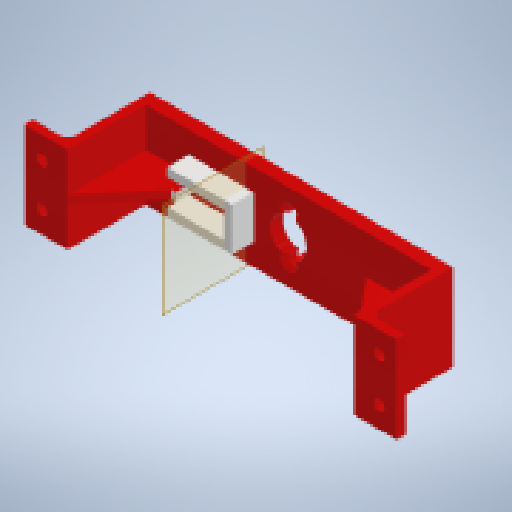
# Autodesk Inventor part: Soporte motor
Saved by Autodesk Inventor 2023 (Build 270158000, 158)
## iProperties
Created: 2022-12-05
Part Number: Soporte motor
Material: Genérico
Document SubType Name: Modeling
Designer: sergi
Density: 1 g/cm^3
Appearance: Valor por defecto
Author: sergi
Autodesk Inventor part; units mm, degrees
ref_plane "XZ Plane" through (0, 0, 0) normal (0, 1, 0) x (-1, 0, 0)
ref_plane "XY Plane" through (0, 0, 0) normal (0, 0, 1) x (1, 0, 0)
sketch "Boceto1" plane through (0, 0, 0) normal (0, 0, 1) x (1, 0, 0)
  circle A0 centre (0, 0) radius 4.25
  line L0 (-35, -10) -> (35, -10)
  line L1 (35, -10) -> (35, 10)
  line L2 (35, 10) -> (-35, 10)
  line L3 (-35, 10) -> (-35, -10)
  line L4 (-35, -10) -> (35, 10) construction
  line L5 (35, -10) -> (-35, 10) construction
  circle A1 centre (0, 0) radius 8
  dimension "d0" = 8.5
  dimension "d1" = 70
  dimension "d2" = 20
  dimension "d3" = 16
  constraints: 12 end point, 2 centre point, 2 coincident, 2 midpoint, 2 parallel, 1 horizontal, 1 perpendicular
  measures "d0" diameter of A0
  measures "d1" distance of L2.end L1.end
  measures "d2" distance of L1.end L0.end
  measures "d3" diameter of A1
extrude "Extrusión1" add sketch "Boceto1" along normal blind 3 contours L3 L2 L1 L0 | A1
sketch "Boceto3" plane through (0, 0, 3) normal (0, 0, 1) x (1, 0, 0)
  line L0 (-35, 10) -> (-35, -10) projected
  line L1 (-35, -10) -> (-33, -10)
  line L2 (-33, -10) -> (-33, 10)
  line L3 (-33, 10) -> (-35, 10)
  line L4 (-35, 10) -> (-35, -10)
  line L5 (35, -10) -> (33, -10)
  line L6 (33, -10) -> (33, 10)
  line L7 (33, 10) -> (35, 10)
  line L8 (35, 10) -> (35, -10)
  point P0 (0, 0)
  dimension "d10" = 2
  dimension "d11" = 20
  dimension "d12" = 2
  dimension "d13" = 20
  constraints: 16 end point, 4 parallel, 2 horizontal, 2 perpendicular, 1 point on line
  measures "d10" distance of L3.end L2.end
  measures "d11" distance of L2.end L1.end
  measures "d12" distance of L6.end L7.end
  measures "d13" distance of L5.end L6.end
ref_plane "Plano de trabajo1" through (-48.5042, -32, 20) normal (0, 0, -1) x (0, 1, 0)
extrude "Extrusión3" add sketch "Boceto3" along normal blind 18
sketch "Boceto4" plane through (0, 0, 3) normal (0, 0, 1) x (1, 0, 0)
  circle A0 centre (0, 0) radius 4.25 projected
  circle A1 centre (0, -5) radius 1 projected
  circle A2 centre (0, 5) radius 1 projected
hole "Agujero1" at (0, -5, 3) at (0, 5, 3) direction (0, 0, -1) diameter 2 depth 3
chamfer "Chaflán1" distance 1 angle 45 2 edges at (0, 6, 3) (0, -6, 3)
sketch "Boceto5" plane through (-35, -10, 0) normal (-1, 0, 0) x (0, 0, 1)
  line L0 (0, 0) -> (21, 0) projected
  line L1 (21, 0) -> (19, 0)
  line L2 (19, 0) -> (19, 20)
  line L3 (19, 20) -> (21, 20)
  line L4 (21, 20) -> (21, 0)
  point P0 (0, 10)
  dimension "d49" = 2
  dimension "d50" = 20
  constraints: 8 end point, 2 parallel, 1 horizontal, 1 perpendicular
  measures "d49" distance of L2.end L3.end
  measures "d50" distance of L1.end L2.end
extrude "Extrusión4" add sketch "Boceto5" along normal blind 8
sketch "Boceto6" plane through (35, -10, 0) normal (1, 0, 0) x (0, 0, -1)
  line L0 (0, 20) -> (-21, 20) projected
  line L1 (-21, 20) -> (-19, 20)
  line L2 (-19, 20) -> (-19, 0)
  line L3 (-19, 0) -> (-21, 0)
  line L4 (-21, 0) -> (-21, 20)
  point P0 (0, 10)
  dimension "d51" = 2
  dimension "d52" = 20
  constraints: 8 end point, 2 parallel, 1 horizontal, 1 perpendicular
  measures "d51" distance of L2.end L3.end
  measures "d52" distance of L1.end L2.end
extrude "Extrusión5" add sketch "Boceto6" along normal blind 8
sketch "Boceto8" plane through (0, 0, 21) normal (0, 0, 1) x (1, 0, 0)
  line L0 (43, 10) -> (43, -10) projected
  line L1 (33, 10) -> (43, 10) projected
  line L2 (33, -10) -> (43, -10) projected
  point P0 (0, 0)
  point P1 (39, -5)
  point P2 (39, 5)
  dimension "d53" = 4
  dimension "d54" = 4
  dimension "d55" = 5
  dimension "d56" = 5
  measures "d53" distance from line of L0 point (39, -5)
  measures "d54" distance from line of L0 point (39, 5)
  measures "d55" distance from line of L1 point (39, 5)
  measures "d56" distance from line of L2 point (39, -5)
hole "Agujero3" at (39, 5, 21) at (39, -5, 21) direction (0, 0, -1) diameter 2.5 end through all
sketch "Boceto9" plane through (0, 0, 21) normal (0, 0, 1) x (1, 0, 0)
  line L0 (-33, 10) -> (-43, 10) projected
  line L1 (-43, -10) -> (-43, 10) projected
  line L2 (-33, -10) -> (-43, -10) projected
  point P0 (0, 0)
  point P1 (-39, 5)
  point P2 (-39, -5)
  dimension "d64" = 5
  dimension "d65" = 4
  dimension "d73" = 5
  dimension "d74" = 4
  measures "d64" distance from line of L0 point (-39, 5)
  measures "d65" distance from line of L1 point (-39, 5)
  measures "d73" distance from line of L2 point (-39, -5)
  measures "d74" distance from line of L1 point (-39, -5)
hole "Agujero4" at (-39, 5, 21) at (-39, -5, 21) direction (0, 0, -1) diameter 2.5 end through all
sketch "Boceto10" plane through (0, 0, 3) normal (0, 0, 1) x (1, 0, 0)
  line L0 (33, -10) -> (33, 10) projected
  line L1 (33, 0) -> (33, 1)
  line L2 (33, 0) -> (34, 0) construction
  line L3 (33, 1) -> (18, 1)
  line L4 (18, 1) -> (18, -1)
  line L5 (18, -1) -> (33, -1)
  line L6 (33, -1) -> (33, 1)
  point P0 (0, 0)
  dimension "d75" = 1
  dimension "d76" = 90
  dimension "d77" = 15
  dimension "d78" = 2
  constraints: 12 end point, 2 horizontal, 2 parallel, 2 perpendicular, 1 collinear, 1 midpoint
  measures "d75" distance of L1.start L1.end
  measures "d76" angle of L2 L1
  measures "d77" distance of L5.end L4.end
  measures "d78" distance of L4.end L3.end
extrude "Extrusión6" add sketch "Boceto10" along normal blind 18
chamfer "Chaflán2" distance 15 distance2 18 1 edges at (18, 0, 21) measured on face at (18.5, 0, 21)
fillet "Empalme2" radius 2 2 edges at (35, 0, 19) (-35, 0, 19)
mirror "Simetría1" about plane through (0, 0, 0) normal (1, 0, 0) of "Extrusión6", "Chaflán2"
ref_plane "Plano de trabajo2" through (-10, 0, 0) normal (1, 0, 0) x (0, 1, 0)
sketch "Boceto12" plane through (0, 0, 3) normal (0, 0, 1) x (1, 0, 0)
  line L0 (-10, -3) -> (-21, -3) projected
  line L1 (-21, -3) -> (-21, 3) projected
  line L2 (-10, 3) -> (-21, 3) projected
  line L3 (-10, -3) -> (-10, 3) projected
  point P0 (0, 0)
extrude "Extrusión7" cut sketch "Boceto12" along normal blind 10
sketch "Boceto13" plane through (0, 0, 3) normal (0, 0, 1) x (1, 0, 0)
  line L0 (-10, -3) -> (-21, -3) projected
  line L1 (-21, -3) -> (-21, 3) projected
  line L2 (-10, 3) -> (-21, 3) projected
  line L3 (-10, -3) -> (-10, 3) projected
  line L4 (-23, -5) -> (-8, -5)
  line L5 (-8, -5) -> (-8, 5)
  line L6 (-8, 5) -> (-23, 5)
  line L7 (-23, 5) -> (-23, -5)
  line L8 (-10, -3) -> (-8, -3)
  line L9 (-10, 3) -> (-8, 3)
  line L10 (-33, -1) -> (-21, -1) projected
  line L11 (-21, 1) -> (-33, 1) projected
  line L12 (-21, -3) -> (-23, -3)
  line L13 (-21, 3) -> (-23, 3)
  point P0 (0, 0)
  point P1 (-23, 1)
  point P2 (-23, -1)
  dimension "d88" = 2
  constraints: 16 end point, 4 point on line, 3 perpendicular, 1 parallel, 3 other
  measures "d88" distance between parallel lines of L0 L4
extrude "Extrusión8" add sketch "Boceto13" along normal blind 5 contours L8 L5 L4 L7 L12 L0 | L3 L9 L5 L8 | L2 L13 L7 L6 L5 L9
sketch "Boceto14" plane through (0, 0, 8) normal (0, 0, 1) x (1, 0, 0)
  line L0 (-10, 3) -> (-10, -3) projected
  line L1 (-10, 3) -> (-23, 3)
  line L2 (-23, 3) -> (-23, -3)
  line L3 (-23, -3) -> (-10, -3)
  line L4 (-10, -3) -> (-10, 3)
  point P0 (0, 0)
  constraints: 8 end point, 2 parallel, 1 horizontal, 1 perpendicular
extrude "Extrusión9" cut sketch "Boceto14" along normal blind 5 and the other way blind 5
